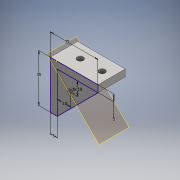
# Autodesk Inventor part: angle_90_profile_2020
Saved by Autodesk Inventor 2016 (Build 200138000, 138)
## iProperties
Created: 2018-10-24
Part Number: angle_90_profile_2020
Material: Generic
Document SubType Name: Modeling
Designer: mbouhier
Density: 1 g/cm^3
Appearance: Default
Author: mbouhier
Autodesk Inventor part; units mm, degrees
ref_plane "YZ Plane" through (0, 0, 0) normal (1, 0, 0) x (0, 1, 0)
ref_plane "XZ Plane" through (0, 0, 0) normal (0, 1, 0) x (-1, 0, 0)
ref_plane "XY Plane" through (0, 0, 0) normal (0, 0, 1) x (1, 0, 0)
sketch "Sketch1" plane through (0, 0, 0) normal (0, 1, 0) x (-1, 0, 0)
  line L0 (0, 0) -> (-35, 0)
  line L1 (-35, 0) -> (-35, -5)
  line L2 (-5, -35) -> (0, -35)
  line L3 (0, -35) -> (0, 0)
  line L4 (-5, -5) -> (-35, -5)
  line L5 (-5, -35) -> (-5, -5)
  line L6 (-35, -5) -> (-5, -35)
  point P0 (-15, -15)
  dimension "d2" = 5
  dimension "d3" = 5
  dimension "d4" = 10
  dimension "d5" = 10
  dimension "d6" = 35
  dimension "d7" = 35
  constraints: 14 end point, 2 horizontal, 2 parallel, 1 perpendicular
  measures "d2" distance between parallel lines of L3 L5
  measures "d3" distance between parallel lines of L4 L0
  measures "d4" distance from line of point (-15, -15) L5
  measures "d5" distance from line of point (-15, -15) L4
  measures "d6" distance of L0.start L0.end
  measures "d7" distance of L2.end L0.start
extrude "Extrusion1" add sketch "Sketch1" along normal blind 20 contours L3 L2 L5 L4 L1 L0
extrude "Extrusion2" add sketch "Sketch1" along normal blind 5 contours L4 L5 L6
sketch "Sketch2" plane through (5, 20, -5) normal (1, 0, 0) x (0, 0, -1)
  point P0 (-5, -20)
ref_plane "Work Plane1" through (5, 20, -5) normal (0.7071, 0, 0.7071) x (0, -1, 0)
sketch "Sketch3" plane through (5, 20, -5) normal (1, 0, 0) x (0, 0, -1)
  line L0 (0, 0) -> (30, 0) projected
  line L1 (0, -15) -> (0, 0) projected
  line L2 (30, -15) -> (30, 0) projected
  point P0 (-5, -20)
  point P1 (7, -10)
  point P2 (23, -10)
  dimension "d12" = 10
  dimension "d13" = 7
  dimension "d14" = 7
  dimension "d15" = 10
  measures "d12" distance from line of point (7, -10) L0
  measures "d13" distance from line of L1 point (7, -10)
  measures "d14" distance from line of point (23, -10) L2
  measures "d15" distance from line of L0 point (23, -10)
sketch "Sketch4" plane through (0, 5, 0) normal (0, 1, 0) x (1, 0, 0)
  point P0 (0, 0)
  point P1 (15, 15)
hole "Hole1" at (15, 5, -15) direction (0, -1, 0) diameter 4.5 end through all counterbore diameter 8 counterbore depth 2
hole "Hole2" at (5, 10, -12) at (5, 10, -28) direction (-1, 0, 0) diameter 4.5 end through all counterbore diameter 8 counterbore depth 2
mirror "Mirror1" about plane through (5, 20, -5) normal (0.7071, 0, 0.7071) of "Hole2"
equation "\"d5\" = d4"
equation "\"d15\" = d12"
body "Solid1"
